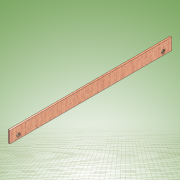
# Autodesk Inventor part: Riel_Lateral_MDF
Saved by Autodesk Inventor 2022 (Build 260153000, 153)
## iProperties
Created: 2022-02-12
Part Number: Riel_Lateral_MDF
Material: Genérico
Document SubType Name: Modeling
Designer: Marco
Density: 1 g/cm^3
Appearance: Abedul - Natural pulido
Author: Marco
Autodesk Inventor part; units mm, degrees
ref_plane "YZ Plane" through (0, 0, 0) normal (1, 0, 0) x (0, 1, 0)
ref_plane "XZ Plane" through (0, 0, 0) normal (0, 1, 0) x (-1, 0, 0)
ref_plane "XY Plane" through (0, 0, 0) normal (0, 0, 1) x (1, 0, 0)
sketch "Boceto1" plane through (0, 0, 0) normal (1, 0, 0) x (0, 1, 0)
  line L0 (0, 0) -> (20, 0)
  line L1 (20, 0) -> (20, -280)
  line L2 (20, -280) -> (0, -280)
  line L3 (0, -280) -> (0, 0)
  circle A0 centre (6, -15) radius 3.175
  circle A1 centre (6, -265) radius 3.175
  dimension "d0" = 20
  dimension "d1" = 280
  dimension "d2" = 6.35
  dimension "d8" = 6
  dimension "d9" = 250
  dimension "d10" = 15
  constraints: 8 end point, 2 centre point, 2 parallel, 1 equal radius, 1 horizontal, 1 perpendicular, 1 vertical alignment
  measures "d0" distance of L1.end L2.end
  measures "d1" distance of L2.end L0.start
  measures "d2" diameter of A0
  measures "d8" horizontal distance of L0.start A0.centre
  measures "d9" distance of A1.centre A0.centre
  measures "d10" vertical distance of L0.start A0.centre
extrude "Extrusión1" add sketch "Boceto1" along normal blind 3
